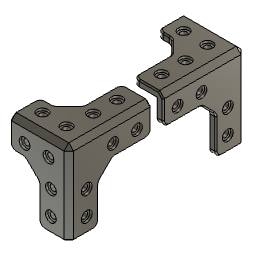
_corner brackets.35f45535-52fe-4c7a-9ea4-c18f3b0c6e2f (Autodesk Fusion 360 design; units mm, degrees)
Autodesk Fusion 360 part; units mm, degrees
sketch "Sketch1" plane through (0, 0, 0) normal (1, 0, 0) x (0, 1, 0)
  line L0 (0, 0) -> (20, 0) construction
  line L1 (20, 0) -> (20, 20) construction
  line L2 (20, 20) -> (0, 20) construction
  line L3 (0, 20) -> (0, 0) construction
  line L4 (20, 20) -> (70, 20) construction
  line L5 (70, 20) -> (70, 0) construction
  line L6 (70, 0) -> (20, 0) construction
  line L7 (20, 0) -> (20, 20) construction
  line L8 (0, 0) -> (20, 0) construction
  line L9 (20, 0) -> (20, -50) construction
  line L10 (20, -50) -> (0, -50) construction
  line L11 (0, -50) -> (0, 0) construction
  line L12 (10, 0) -> (10, -50) construction
  line L13 (20, 10) -> (70, 10) construction
  circle A0 centre (10, -12) radius 2.65
  circle A1 centre (10, -32) radius 2.65
  circle A2 centre (32, 10) radius 2.65
  circle A3 centre (52, 10) radius 2.65
  line L14 (0, -44) -> (20, -44)
  line L15 (20, -44) -> (20, -12)
  line L16 (20, -12) -> (32, 0)
  line L17 (32, 0) -> (64, 0)
  line L18 (64, 20) -> (64, 0)
  line L19 (64, 20) -> (64, 25)
  line L20 (64, 25) -> (0, 25)
  line L21 (0, 25) -> (-5, 25)
  line L22 (-5, 25) -> (-5, -44)
  line L23 (-5, -44) -> (0, -44)
  line L24 (0, -44) -> (0, 25)
  line L25 (64, 20) -> (-5, 20)
  point P0 (20, -12)
  point P1 (32, 0)
  dimension "d1" = 20
  dimension "d2" = 20
  dimension "d3" = 50
  dimension "d4" = 50
  dimension "d5" = 20
  dimension "d6" = 5.3
  dimension "d7" = 12
  dimension "d8" = 5.3
  dimension "d9" = 20
  dimension "d10" = 5.3
  dimension "d11" = 5.3
  dimension "d12" = 12
  dimension "d13" = 20
  dimension "d14" = 12
  dimension "d15" = 12
  dimension "d16" = 12
  dimension "d17" = 12
  dimension "d18" = 5
  dimension "d19" = 5
  constraint horizontal L0
  constraint vertical L1
  constraint horizontal L2
  constraint vertical L3
  constraint coincident L0.start L3.end
  constraint horizontal L4
  constraint vertical L5
  constraint horizontal L6
  constraint vertical L7
  constraint horizontal L8
  constraint vertical L9
  constraint horizontal L10
  constraint vertical L11
  constraint midpoint L0 L12.start
  constraint midpoint L10 L12.end
  constraint perpendicular L10 L12
  constraint midpoint L7 L13.start
  constraint midpoint L5 L13.end
  constraint coincident L12 A0.centre
  constraint coincident L12 A1.centre
  constraint coincident L13 A2.centre
  constraint coincident L13 A3.centre
  constraint coincident L9 P0
  constraint coincident L6 P1
  constraint coincident L11 L14.start
  constraint coincident L9 L14.end
  constraint perpendicular L9 L14
  constraint coincident P0 L15.end
  constraint coincident P1 L16.end
  constraint coincident L6 L17.end
  constraint perpendicular L9 L17
  constraint coincident L4 L18.start
  constraint perpendicular L6 L18
  constraint perpendicular L4 L19
  constraint perpendicular L3 L20
  constraint perpendicular L3 L21
  constraint perpendicular L14 L22
  constraint perpendicular L11 L23
  constraint perpendicular L21 L24
  constraint coincident L22 L25.end
  constraint perpendicular L22 L25
  measures "d1" distance of L0.start L0.end
  measures "d2" distance of L0.start L2.end
  measures "d3" distance of L1.end L4.end
  measures "d4" distance of L0.start L10.end
  measures "d5" distance of L4 L6
  measures "d6" diameter of A0
  measures "d7" distance of L12.start A0.centre
  measures "d8" diameter of A1
  measures "d9" distance of A0.centre A1.centre
  measures "d10" diameter of A2
  measures "d11" diameter of A3
  measures "d12" distance of L1 A2.centre
  measures "d13" distance of A2.centre A3.centre
  measures "d14" distance of L0.end P1
  measures "d15" distance of L0.end P0
  measures "d16" distance of A1.centre L14
  measures "d17" distance of A3.centre L18
  measures "d18" distance of L18.start L19.end
  measures "d19" distance of L20.end L21.end
extrude "Extrude1" add sketch "Sketch1" along normal blind 5 makes body 1
ref_plane "WorkPlane1" through (2.5, 29.5, 20) normal (0, 0, 1) x (0, -1, 0)
sketch "Sketch2" plane through (0, 0, 20) normal (0, 0, 1) x (1, 0, 0)
  line L0 (0, 0) -> (-50, 0) construction
  line L1 (-50, 0) -> (-50, 20) construction
  line L2 (-50, 20) -> (0, 20) construction
  line L3 (0, 20) -> (0, 0) construction
  line L4 (0, 10) -> (-50, 10) construction
  circle A0 centre (-12, 10) radius 2.65
  circle A1 centre (-32, 10) radius 2.65
  line L5 (0, 64) -> (0, 0) construction
  line L6 (0, 20) -> (-44, 20)
  line L7 (-44, 0) -> (-44, 20)
  line L8 (-44, 0) -> (-44, -5)
  line L9 (-44, -5) -> (0, -5)
  line L10 (0, -5) -> (0, 0)
  line L11 (0, 0) -> (-44, 0)
  line L12 (0, 20) -> (-20, 20)
  line L13 (-20, 20) -> (-20, 64)
  line L14 (-20, 64) -> (0, 64)
  line L15 (0, 64) -> (0, 20)
  line L16 (-10, 20) -> (-10, 64) construction
  circle A2 centre (-10, 30.4164) radius 2.65
  circle A3 centre (-10, 50.4164) radius 2.65
  line L17 (0, 20) -> (0, 0)
  line L18 (-32, 20) -> (-20, 32)
  point P0 (0, 20)
  point P1 (0, 64)
  dimension "d23" = 50
  dimension "d24" = 20
  dimension "d25" = 5.3
  dimension "d26" = 5.3
  dimension "d27" = 20
  dimension "d28" = 12
  dimension "d29" = 5
  dimension "d30" = 12
  dimension "d31" = 20
  dimension "d32" = 44
  dimension "d33" = 5.3
  dimension "d34" = 5.3
  dimension "d35" = 20
  dimension "d36" = 12
  dimension "d37" = 12
  constraint horizontal L0
  constraint vertical L1
  constraint horizontal L2
  constraint vertical L3
  constraint coincident L0.start L3.end
  constraint midpoint L3 L4.start
  constraint midpoint L1 L4.end
  constraint coincident L4 A0.centre
  constraint coincident L4 A1.centre
  constraint coincident L2 L6.end
  constraint perpendicular L3 L6
  constraint coincident L0 L7.start
  constraint perpendicular L6 L7
  constraint perpendicular L0 L8
  constraint perpendicular L3 L9
  constraint perpendicular L0 L10
  constraint horizontal L12
  constraint vertical L13
  constraint horizontal L14
  constraint vertical L15
  constraint midpoint L12 L16.start
  constraint midpoint L14 L16.end
  constraint coincident L16 A2.centre
  constraint coincident L16 A3.centre
  constraint coincident P0 L2.end
  constraint coincident L2 L18.start
  constraint coincident L13 L18.end
  measures "d23" distance of L0.start L0.end
  measures "d24" distance of L0.start P0
  measures "d25" diameter of A0
  measures "d26" diameter of A1
  measures "d27" distance of A0.centre A1.centre
  measures "d28" distance of A0.centre L5
  measures "d29" distance of L7.start L8.end
  measures "d30" distance of A1.centre L7
  measures "d31" distance of P0 L12.end
  measures "d32" distance of P0 P1
  measures "d33" diameter of A2
  measures "d34" diameter of A3
  measures "d35" distance of A2.centre A3.centre
  measures "d36" distance of L12.end L18.start
  measures "d37" distance of L12.end L18.end
extrude "Extrude2" add sketch "Sketch2" along normal blind 5 bodies 1
ref_plane "WorkPlane2" through (-19.5, 0, -9.5) normal (0, -1, 0) x (0, 0, -1)
sketch "Sketch3" plane through (0, 0, 0) normal (0, -1, 0) x (-1, 0, 0)
  line L0 (44, -20) -> (0, -20)
  line L1 (0, -25) -> (0, 44)
  line L2 (0, -20) -> (20, -20)
  line L3 (20, -20) -> (20, 0)
  line L4 (20, 0) -> (0, 0)
  line L5 (0, 0) -> (0, -20)
  line L6 (20, 0) -> (0, 0)
  line L7 (0, 0) -> (0, 44)
  line L8 (0, 44) -> (20, 44)
  line L9 (20, 44) -> (20, 0)
  line L10 (20, -20) -> (44, -20)
  line L11 (44, -20) -> (44, 0)
  line L12 (44, 0) -> (20, 0)
  line L13 (20, 0) -> (20, -20)
  line L14 (32, 0) -> (20, 12)
  line L15 (10, 0) -> (10, 44) construction
  circle A0 centre (10, 12) radius 2.65
  circle A1 centre (10, 32) radius 2.65
  line L16 (44, -10) -> (0, -10) construction
  circle A2 centre (12, -10) radius 2.65
  circle A3 centre (32, -10) radius 2.65
  dimension "d41" = 20
  dimension "d42" = 20
  dimension "d43" = 12
  dimension "d44" = 12
  dimension "d45" = 5.3
  dimension "d46" = 5.3
  dimension "d47" = 20
  dimension "d48" = 12
  dimension "d49" = 5.3
  dimension "d50" = 5.3
  dimension "d51" = 20
  dimension "d52" = 12
  constraint horizontal L2
  constraint vertical L3
  constraint horizontal L4
  constraint vertical L5
  constraint coincident L0.end L2.start
  constraint horizontal L6
  constraint vertical L7
  constraint horizontal L8
  constraint vertical L9
  constraint coincident L1.end L7.end
  constraint horizontal L10
  constraint vertical L11
  constraint horizontal L12
  constraint vertical L13
  constraint coincident L12 L14.start
  constraint coincident L9 L14.end
  constraint midpoint L6 L15.start
  constraint midpoint L8 L15.end
  constraint coincident L15 A0.centre
  constraint coincident L15 A1.centre
  constraint midpoint L11 L16.start
  constraint midpoint L5 L16.end
  constraint perpendicular L1 L16
  constraint coincident L16 A2.centre
  constraint coincident L16 A3.centre
  measures "d41" distance of L0.end L2.end
  measures "d42" distance of L0.end L4.end
  measures "d43" distance of L3.end L14.end
  measures "d44" distance of L3.end L14.start
  measures "d45" diameter of A0
  measures "d46" diameter of A1
  measures "d47" distance of A0.centre A1.centre
  measures "d48" distance of L4 A0.centre
  measures "d49" diameter of A2
  measures "d50" diameter of A3
  measures "d51" distance of A2.centre A3.centre
  measures "d52" distance of L1 A2.centre
extrude "Extrude3" add sketch "Sketch3" along normal blind 5 bodies 1
chamfer "Chamfer1" distance 4 angle 45 3 edges at (5, -5, -9.5) (5, 29.5, 25) (-19.5, -5, 25) on bodies 1
sketch "Sketch4" plane through (0, 0, 25) normal (0, 0, 1) x (-1, 0, 0)
  circle A0 centre (12, -10) radius 2.65 construction
  circle A1 centre (32, -10) radius 2.65 construction
  circle A2 centre (10, -30.4164) radius 2.65 construction
  circle A3 centre (10, -50.4164) radius 2.65 construction
  circle A4 centre (32, -10) radius 4.5
  circle A5 centre (12, -10) radius 4.5
  circle A6 centre (10, -30.4164) radius 4.5
  circle A7 centre (10, -50.4164) radius 4.5
  dimension "d56" = 9
  dimension "d57" = 9
  dimension "d58" = 9
  dimension "d59" = 9
  constraint concentric A1 A4
  constraint concentric A0 A5
  constraint concentric A2 A6
  constraint concentric A3 A7
  measures "d56" diameter of A4
  measures "d57" diameter of A5
  measures "d58" diameter of A6
  measures "d59" diameter of A7
extrude "Extrude4" cut sketch "Sketch4" against normal blind 2 bodies 1
sketch "Sketch5" plane through (5, 0, 0) normal (1, 0, 0) x (0, 1, 0)
  circle A0 centre (32, 10) radius 2.65 construction
  circle A1 centre (52, 10) radius 2.65 construction
  circle A2 centre (10, -12) radius 2.65 construction
  circle A3 centre (10, -32) radius 2.65 construction
  circle A4 centre (10, -32) radius 4.5
  circle A5 centre (10, -12) radius 4.5
  circle A6 centre (32, 10) radius 4.5
  circle A7 centre (52, 10) radius 4.5
  dimension "d62" = 9
  dimension "d63" = 9
  dimension "d64" = 9
  dimension "d65" = 9
  constraint concentric A3 A4
  constraint concentric A2 A5
  constraint concentric A0 A6
  constraint concentric A1 A7
  measures "d62" diameter of A4
  measures "d63" diameter of A5
  measures "d64" diameter of A6
  measures "d65" diameter of A7
extrude "Extrude5" cut sketch "Sketch5" against normal blind 2 bodies 1
sketch "Sketch6" plane through (0, -5, 0) normal (0, -1, 0) x (1, 0, 0)
  circle A0 centre (-12, 10) radius 2.65 construction
  circle A1 centre (-32, 10) radius 2.65 construction
  circle A2 centre (-10, -12) radius 2.65 construction
  circle A3 centre (-10, -32) radius 2.65 construction
  circle A4 centre (-12, 10) radius 4.5
  circle A5 centre (-32, 10) radius 4.5
  circle A6 centre (-10, -12) radius 4.5
  circle A7 centre (-10, -32) radius 4.5
  dimension "d68" = 9
  dimension "d69" = 9
  dimension "d70" = 9
  dimension "d71" = 9
  constraint concentric A0 A4
  constraint concentric A1 A5
  constraint concentric A2 A6
  constraint concentric A3 A7
  measures "d68" diameter of A4
  measures "d69" diameter of A5
  measures "d70" diameter of A6
  measures "d71" diameter of A7
extrude "Extrude6" cut sketch "Sketch6" against normal blind 2 bodies 1
fillet "Fillet1" radius 5 12 edges at (2.5, 64, 0) (2.5, 20, -44) (2.5, 20, -12) (2.5, 32, 0) (-20, -2.5, -44) (-20, -2.5, -12) (-32, -2.5, 0) (-44, -2.5, 0) (-44, 20, 22.5) (-32, 20, 22.5) (-20, 32, 22.5) (-20, 64, 22.5) on bodies 1
chamfer "Chamfer2" distance 1 angle 45 30 edges at (5, 7, -44) (5, 18.5355, -42.5355) (5, 20, -26.5355) (5, 20.3806, -12.1577) (5, 26, -6) (5, 32.1577, -0.3806) (5, 46.5355, 0) (5, 62.5355, 1.4645) (5, 64, 13) (3, -3, -44) (-7, -5, -44) (-44, -5, 13) (-42.5355, -5, 1.4645) (-36.5355, -5, 0) (-32.1577, -5, -0.3806) (-26, -5, -6) (-20.3806, -5, -12.1577) (-20, -5, -26.5355) (-18.5355, -5, -42.5355) (3, 64, 23) (-7, 64, 25) (-44, 7, 25) (-42.5355, 18.5355, 25) (-36.5355, 20, 25) (-32.1577, 20.3806, 25) (-26, 26, 25) (-20.3806, 32.1577, 25) (-20, 46.5355, 25) (-18.5355, 62.5355, 25) (-44, -3, 23) on bodies 1
mirror "Mirror1" about plane through (0, 64, 20) normal (0, 1, 0) of bodies 1 makes body 2
move_body "Move1" bodies 2 to x (1, 0, 0) y (0, 1, 0) z (0, 0, 1) at (0, 10, 0)
equation "d32 = 20 mm + 12 mm + 12 mm"
